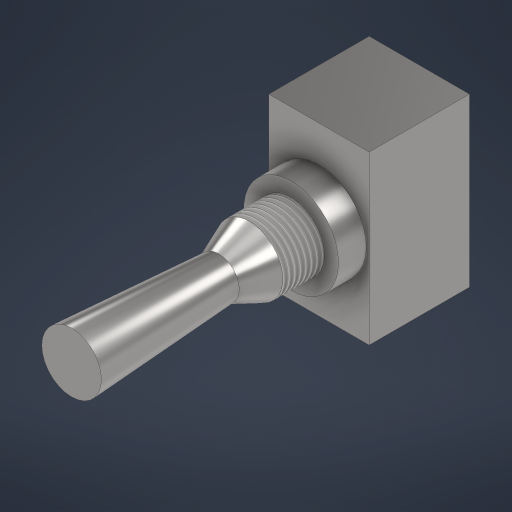
# Autodesk Inventor part: NKK_S1AL
Saved by Autodesk Inventor 2024 (Build 280153000, 153)
## iProperties
Created: 2026-04-07
Part Number: NKK_S1AL
Material: Stainless Steel
Document SubType Name: Modeling
Designer: schar
Density: 8 g/cm^3
Appearance: Semi-Polished
Author: schar
Autodesk Inventor part; units mm, degrees
ref_plane "YZ Plane" through (0, 0, 0) normal (1, 0, 0) x (0, 1, 0)
ref_plane "XZ Plane" through (0, 0, 0) normal (0, 1, 0) x (-1, 0, 0)
sketch "Sketch1" plane through (0, 0, 0) normal (1, 0, 0) x (0, 1, 0)
  point P0 (0, 0)
sketch "Sketch2" plane through (0, 0, 0) normal (1, 0, 0) x (0, 1, 0)
  line L0 (15, 9) -> (-15, 9)
  line L1 (-15, 9) -> (-15, -9)
  line L2 (-15, -9) -> (15, -9)
  line L3 (15, -9) -> (15, 9)
  line L4 (15, 9) -> (-15, -9) construction
  line L5 (-15, 9) -> (15, -9) construction
  point P0 (0, 0)
  dimension "d0" = 30
  dimension "d1" = 18
  constraints: 12 end point, 2 midpoint, 2 parallel, 1 horizontal, 1 perpendicular
  measures "d0" distance of L2.end L1.end
  measures "d1" distance of L1.end L0.end
extrude "Extrusion1" add sketch "Sketch2" along normal blind 18
sketch "Sketch3" plane through (0, -15, 9) normal (0, 0, 1) x (1, 0, 0)
  line L0 (18, 0) -> (18, 30) projected
  line L1 (0, 0) -> (0, 30) projected
  line L2 (18, 0) -> (0, 30)
  line L3 (0, 0) -> (18, 0) projected
  line L4 (0, 30) -> (0, 0)
  line L5 (0, 0) -> (18, 30)
  circle A0 centre (9, 15) radius 8.5
  point P0 (0, 15)
  dimension "d4" = 17
  constraints: 6 end point, 1 centre point, 1 midpoint, 1 perpendicular
  measures "d4" diameter of A0
extrude "Extrusion2" add sketch "Sketch3" along normal blind 5 contours A0 L5 L2 | L2 L5 A0 | L5 L2 A0 | L5 A0 L2
sketch "Sketch4" plane through (9, 0, 14) normal (0, 0, 1) x (1, 0, 0)
  circle A0 centre (0, 0) radius 6
  point P0 (-9, 0)
  dimension "d7" = 12
  constraints: 1 centre point
  measures "d7" diameter of A0
extrude "Extrusion3" add sketch "Sketch4" along normal blind 7.5
sketch "Sketch5" plane through (9, 0, 21.5) normal (0, 0, 1) x (1, 0, 0)
  circle A0 centre (0, 0) radius 6
  point P0 (-9, 0)
  constraints: 1 centre point
extrude "Extrusion4" add sketch "Sketch5" along normal blind 5.5
sketch "Sketch6" plane through (0, 0, 0) normal (1, 0, 0) x (0, 1, 0)
  point P0 (0, 0)
ref_plane "Work Plane1" through (9, 0, 0) normal (1, 0, 0) x (0, 0, -1)
sketch "Sketch7" plane through (9, 0, 0) normal (1, 0, 0) x (0, 0, -1)
  line L0 (-27, 6) -> (-27, -6) projected
  line L1 (-27, 0) -> (-27, 3.7)
  line L2 (-27, 0) -> (-27, -3.7)
  line L3 (-14, -6) -> (-14, 6) projected
  line L4 (-14, -6) -> (-21.5, -6)
  line L5 (-14, -6) -> (-27, -6) projected
  line L6 (-21.5, -6) -> (-27, -3.7)
  line L7 (-27, -6) -> (-27, -3.7)
  line L8 (-21.5, -6) -> (-27, -6)
  line L9 (-40.6184, 0) -> (-19.5493, 0)
  point P0 (0, 0)
  dimension "d12" = 3.7
  dimension "d13" = 3.7
  dimension "d14" = 7.5
  constraints: 14 end point, 4 point on line, 2 collinear, 1 coincident, 1 horizontal, 1 midpoint
  measures "d12" distance of L1.start L1.end
  measures "d13" distance of L1.start L2.end
  measures "d14" distance of L3.start L4.end
revolve "Revolution1" cut sketch "Sketch7" angle 360 about axis through (9, 0, 40.6184) along (0, 0, -1)
sketch "Sketch8" plane through (9, 0, 27) normal (0, 0, 1) x (1, 0, 0)
  circle A0 centre (0, 0) radius 3.7 projected
  circle A1 centre (0, 0) radius 5.35
  point P0 (-9, 0)
  dimension "d16" = 10.7
  constraints: 1 centre point, 1 coincident
  measures "d16" diameter of A1
extrude "Extrusion5" add sketch "Sketch8" along normal blind 26.4 contours A0 | A1
sketch "Sketch9" plane through (9, 0, 0) normal (1, 0, 0) x (0, 0, -1)
  line L0 (-27, 3.7) -> (-27, -3.7) projected
  line L1 (-27, 3.7) -> (-53.4, 5.35)
  line L2 (-27, 5.35) -> (-53.4, 5.35) projected
  line L3 (-27, 3.7) -> (-27, 5.35)
  line L4 (-66.1655, 0) -> (-43.0091, 0)
  line L5 (-53.4, 5.35) -> (-53.4, -5.35) projected
  point P0 (0, 0)
  point P1 (-53.4, 0)
  constraints: 6 end point, 2 point on line, 1 horizontal, 1 midpoint, 1 vertical
revolve "Revolution2" cut sketch "Sketch9" angle 360 about axis through (9, 0, 66.1655) along (0, 0, -1)
thread "Thread1" size "M12x1" class "6g" standard "ANSI Metric M Profile" length 15.103
body "Solid1"
